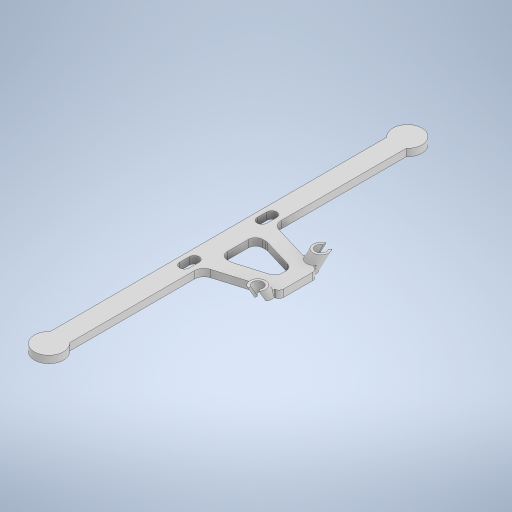
# Autodesk Inventor part: supporto_marker
Saved by Autodesk Inventor 2023.2 (Build 272271030, 271C)
## iProperties
Created: 2023-10-30
Part Number: supporto_marker
Material: Generic
Document SubType Name: Modeling
Designer: matti
Density: 1 g/cm^3
Appearance: Default
Author: matti
Autodesk Inventor part; units mm, degrees
ref_plane "YZ Plane" through (0, 0, 0) normal (1, 0, 0) x (0, 1, 0)
ref_plane "XZ Plane" through (0, 0, 0) normal (0, 1, 0) x (-1, 0, 0)
sketch "Sketch1" plane through (0, 0, 0) normal (0, 1, 0) x (-1, 0, 0)
  line L0 (13.0634, 0) -> (-36.3807, 0) projected
  line L1 (0, -112) -> (0, 112) projected
  circle A0 centre (0, 74) radius 6
  circle A1 centre (0, -74) radius 6
  line L2 (4, -69.5279) -> (4, 69.5279)
  line L3 (-4, 69.5279) -> (-4, -69.5279)
  arc A2 (2, 18) -> (-2, 18) centre (0, 18) ccw
  arc A3 (-2, 14) -> (2, 14) centre (0, 14) ccw
  line L4 (2, 18) -> (2, 14)
  line L5 (-2, 14) -> (-2, 18)
  arc A4 (-2, -18) -> (2, -18) centre (0, -18) ccw
  arc A5 (2, -14) -> (-2, -14) centre (0, -14) ccw
  line L6 (2, -18) -> (2, -14)
  line L7 (-2, -14) -> (-2, -18)
  line L8 (-4, 0) -> (-4, 15)
  line L9 (-29, 0) -> (-29, 6.0119)
  line L10 (-27.5747, 7.9276) -> (-4, 15)
  line L11 (-29, 0) -> (-29, -6.0119)
  line L12 (-27.5747, -7.9276) -> (-4, -15)
  circle A6 centre (-24.0549, 8.9835) radius 3.2
  circle A7 centre (-24.0549, 8.9835) radius 2.2
  circle A8 centre (-24.0549, -8.9835) radius 3.2
  circle A9 centre (-24.0549, -8.9835) radius 2.2
  arc A10 (-27.5747, 7.9276) -> (-29, 6.0119) centre (-27, 6.0119) ccw
  arc A11 (-29, -6.0119) -> (-27.5747, -7.9276) centre (-27, -6.0119) ccw
  line L13 (-4, 15) -> (-4, -15)
  line L14 (-8.7127, 7.322) -> (-23, 3.0358)
  line L15 (-23, 3.0358) -> (-23, 0)
  line L16 (-23, 0) -> (-23, -3.0358)
  line L17 (-23, -3.0358) -> (-8.7127, -7.322)
  line L18 (-8.7127, 7.322) -> (-4, 7.322)
  line L19 (-8.7127, -7.322) -> (-4, -7.322)
  point P0 (0, 0)
  point P1 (0, 16)
  point P2 (-29, 7.5)
  point P3 (-29, -7.5)
  point P4 (-4, 7.322)
  point P5 (-4, -7.322)
  point P6 (-20.9899, 9.903)
  point P7 (-27.12, 8.064)
  point P8 (-27.12, -8.064)
  point P9 (-20.9899, -9.903)
  point P10 (-4, -15)
  dimension "d35" = 70
  dimension "d2" = 12
  dimension "d5" = 16
  dimension "d9" = 15
  dimension "d11" = 7.5
  dimension "d12" = 6.4
  dimension "d13" = 4.4
  dimension "d14" = 2
  dimension "d15" = 6
  constraints: 36 end point, 16 point on circle, 13 point on line, 12 centre point, 11 symmetric about line, 7 tangent, 2 coincident, 2 perpendicular, 1 collinear, 1 equal radius, 1 midpoint, 1 parallel, 8 other
  measures "d2" diameter of A0
  measures "d5" distance of point (0, 16) point (0, 0)
  measures "d9" distance of L8.start L8.end
  measures "d11" distance of L9.start point (-29, 7.5)
  measures "d12" diameter of A6
  measures "d13" diameter of A7
  measures "d14" radius of A10
  measures "d15" distance between parallel lines of L10 L14
extrude "Extrusion1" add sketch "Sketch1" along normal blind 3 contours L3 A0 L1 A2 L5 A3 L0 | L0 L1 A5 L7 A4 A1 L3 | L16 L17 L19 L3 L12 A8 A11 L11 L0 | L0 L9 A10 L10 A6 L3 L18 L14 L15 | L1 A3 L4 A2 A0 L2 L0 | L0 L2 A1 L1 A4 L6 A5 | A1 L1 | A0 L1 | A0 L1 | A1 L1 | A8 L12 A9 | L12 A9 A8 | A9 L12 | L12 A9
fillet "Fillet1" radius 4 1 edges at (4, 1.5, -15)
fillet "Fillet2" radius 4 1 edges at (4, 1.5, 15)
fillet "Fillet3" radius 3 6 edges at (4, 1.5, -7.322) (4, 1.5, 7.322) (23, 1.5, -3.0358) (23, 1.5, 3.0358) (8.7127, 1.5, -7.322) (8.7127, 1.5, 7.322)
ref_plane "Work Plane2" through (24.0549, 0, -8.9835) normal (-0.9578263, 0, -0.2873479) x (0, -1, 0)
sketch "Sketch4" plane through (24.0549, 0, -8.9835) normal (-0.9578263, 0, -0.2873479) x (0, -1, 0)
  line L0 (0, -49.9294) -> (0, 83.2618) projected
  line L1 (0, -0.4025) -> (-6.0243, -4.6207)
  line L2 (0, -0.4025) -> (7.3543, -0.4025) construction
  point P0 (0, 15.5168)
  dimension "d25" = 145
  constraints: 4 end point, 1 equal length, 1 horizontal, 1 point on line
  measures "d25" angle of L1 L2
sweep "Sweep1" add profiles "Sketch1" path "Sketch4" path curves L1 contours A8 L12 A9 | L12 A9 A8
sweep "Sweep2" cut profiles "Sketch1" path "Sketch4" path curves L1 contours A9 L12 | L12 A9
sketch "Sketch5" plane through (25.267, 6.0243, -13.0239) normal (0, 1, 0) x (1, 0, 0)
  line L0 (-37.5699, -125.233) -> (28.1273, 93.7578) projected
  circle A0 centre (0, 0) radius 3.2 projected
  line L1 (0.9195, 3.065) -> (-0.9961, 3.6397)
  line L2 (0.9195, 3.065) -> (2.8352, 2.4903)
  line L3 (2.8352, 2.4903) -> (1.8576, 1.1788)
  circle A1 centre (0, 0) radius 2.2 projected
  line L4 (-0.9961, 3.6397) -> (-0.902, 2.0066)
  arc A2 (1.8576, 1.1788) -> (-0.902, 2.0066) centre (0, 0) ccw
  point P0 (-25.267, -13.0239)
  point P1 (-0.902, 2.0066)
  dimension "d33" = 2
  dimension "d34" = 2
  dimension "d35" = 70
  constraints: 8 end point, 2 point on circle, 2 point on line, 1 centre point, 1 coincident, 1 symmetric about line, 6 other
  measures "d33" distance of L1.start L1.end
  measures "d34" distance of L1.start L2.end
  measures "d35" angle of L2 L3
sweep "Sweep3" cut profiles "Sketch5" path "Sketch4" picked at (0.6157, 2.7862) picked at (1.0196, 2.665) path curves L1 contours L4 L1 A0 | A0 L0 A1 L4 | L0 A0 L3 A1 | L2 L3 A0
mirror "Mirror5" about plane through (0, 0, 0) normal (0, 0, 1)
body "Solid1"
